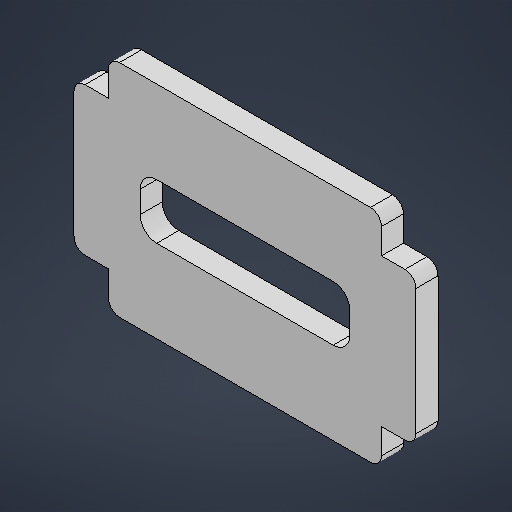
# Autodesk Inventor part: top
Saved by Autodesk Inventor 2026 (Build 300175050, 175E)
## iProperties
Created: 2025-09-02
Part Number: top
Material: 一般
Document SubType Name: Modeling
Designer: ka0n7
Density: 1 g/cm^3
Appearance: 既定
Author: ka0n7
Autodesk Inventor part; units mm, degrees
ref_plane "YZ Plane" through (0, 0, 0) normal (1, 0, 0) x (0, 1, 0)
ref_plane "XZ Plane" through (0, 0, 0) normal (0, 1, 0) x (-1, 0, 0)
ref_plane "XY Plane" through (0, 0, 0) normal (0, 0, 1) x (1, 0, 0)
sketch "スケッチ1" plane through (0, 0, 0) normal (0, 0, 1) x (1, 0, 0)
  line L0 (-24.75, 20) -> (24.75, 20)
  line L1 (24.75, 20) -> (24.75, -20)
  line L2 (24.75, -20) -> (-24.75, -20)
  line L3 (-24.75, -20) -> (-24.75, 20)
  line L4 (-24.75, 20) -> (24.75, -20) construction
  line L5 (24.75, 20) -> (-24.75, -20) construction
  line L6 (-31, 13.4) -> (31, 13.4)
  line L7 (31, 13.4) -> (31, -13.4)
  line L8 (31, -13.4) -> (-31, -13.4)
  line L9 (-31, -13.4) -> (-31, 13.4)
  line L10 (-31, 13.4) -> (31, -13.4) construction
  line L11 (31, 13.4) -> (-31, -13.4) construction
  line L12 (-19, 5) -> (19, 5)
  line L13 (19, 5) -> (19, -5)
  line L14 (19, -5) -> (-19, -5)
  line L15 (-19, -5) -> (-19, 5)
  line L16 (-19, 5) -> (19, -5) construction
  line L17 (19, 5) -> (-19, -5) construction
  point P0 (0, 0)
  point P1 (-24.75, 13.4)
  point P2 (-24.75, -13.4)
  point P3 (24.75, -13.4)
  point P4 (24.75, 13.4)
  dimension "d0" = 49.5
  dimension "d1" = 40
  dimension "d2" = 62
  dimension "d3" = 26.8
  dimension "d4" = 38
  dimension "d5" = 10
  constraints: 36 end point, 6 midpoint, 6 parallel, 3 horizontal, 3 perpendicular
  measures "d0" distance of L1.end L2.end
  measures "d1" distance of L0.end L1.end
  measures "d2" distance of L7.end L8.end
  measures "d3" distance of L6.end L7.end
  measures "d4" distance of L13.end L14.end
  measures "d5" distance of L12.end L13.end
extrude "押し出し1" add sketch "スケッチ1" along normal blind 4
fillet "フィレット1" radius 3 4 edges at (-19, 5, 2) (19, 5, 2) (-19, -5, 2) (19, -5, 2)
fillet "フィレット2" radius 2 8 edges at (24.75, 20, 2) (31, 13.4, 2) (31, -13.4, 2) (24.75, -20, 2) (-24.75, 20, 2) (-31, 13.4, 2) (-31, -13.4, 2) (-24.75, -20, 2)
